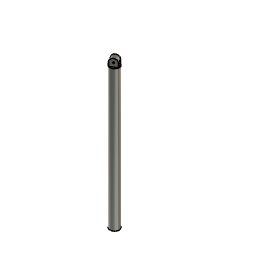
Tripod3 v1 (Autodesk Fusion 360 design; units mm, degrees)
Autodesk Fusion 360 part; units mm, degrees
sketch "Sketch1" plane through (-3, 5.1962, 0) normal (0.5, -0.866025, 0) x (0.866025, 0.5, 0)
  arc A0 (-70.01, 5) -> (-65.01, 0) centre (-65.01, 5) ccw
  line L0 (-65.01, 0) -> (-40.5586, 0)
  line L1 (-40.5586, 0) -> (-40.5586, 16)
  line L2 (-40.5586, 16) -> (-70.01, 16)
  line L3 (-70.01, 16) -> (-70.01, 5)
  circle A1 centre (-60.01, 8) radius 1.6
  arc A2 (-52.21, 8) -> (-67.81, 8) centre (-60.01, 8) ccw
  line L4 (-52.21, 8) -> (-52.21, -0.2)
  line L5 (-52.21, -0.2) -> (-67.81, -0.2)
  line L6 (-67.81, -0.2) -> (-67.81, 8)
  point P0 (-60.01, 8)
  dimension "d46" = 7.8
  dimension "d47" = 8.2
  dimension "d48" = 15.6
  constraint coincident P0 A1.centre
  constraint vertical L4
  constraint horizontal L5
  constraint vertical L6
  measures "d46" radius of A2
  measures "d47" distance of P0 L5
  measures "d48" distance of L4 L6
extrude "Extrude1" add sketch "Sketch1" along normal blind 11.8 contours A0 L0 A2 L4 L6 | A0 L0 L4 L5 L6 makes body 1
sketch "Sketch2" plane through (0, 0, -0.2) normal (0, 0, -1) x (1, 0, 0)
  line L0 (-61.7252, 28.7088) -> (-48.2152, 20.9088)
  line L1 (-48.2152, 20.9088) -> (-42.3152, 31.1279)
  line L2 (-42.3152, 31.1279) -> (-55.8252, 38.9279)
  line L3 (-55.8252, 38.9279) -> (-61.7252, 28.7088)
  circle A0 centre (-52.0202, 29.9184) radius 9.9
  circle A1 centre (-52.0202, 29.9184) radius 5.9
  point P0 (-52.0202, 29.9184)
  dimension "d51" = 5.9
  dimension "d52" = 7.8
  dimension "d53" = 19.8
  dimension "d54" = 11.8
  constraint coincident P0 A0.centre
  constraint concentric A0 A1
  measures "d51" distance of L2 P0
  measures "d52" distance of L3 P0
  measures "d53" diameter of A0
  measures "d54" diameter of A1
extrude "Extrude2" add sketch "Sketch2" along normal blind 300 separate body contours L0 L2 L3 A1 | L0 L1 L2 A1 | A0 makes body 2
